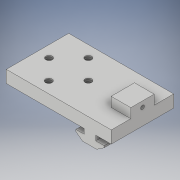
# Autodesk Inventor part: Sliderfor2020
Saved by Autodesk Inventor 2017 (Build 210142000, 142)
## iProperties
Created: 2017-12-08
Part Number: Sliderfor2020
Material: Generic
Document SubType Name: Modeling
Designer: User
Density: 1 g/cm^3
Appearance: Default
Author: User
Autodesk Inventor part; units mm, degrees
ref_plane "YZ Plane" through (0, 0, 0) normal (1, 0, 0) x (0, 1, 0)
ref_plane "XZ Plane" through (0, 0, 0) normal (0, 1, 0) x (-1, 0, 0)
ref_plane "XY Plane" through (0, 0, 0) normal (0, 0, 1) x (1, 0, 0)
sketch "Sketch1" plane through (0, 0, 0) normal (0, 0, 1) x (1, 0, 0)
  line L0 (0, 0) -> (14.5304, 0)
  line L1 (-8.7854, 6.6412) -> (8.5466, 6.6412)
  line L2 (8.5466, 1.6412) -> (2.2606, 1.6412)
  line L3 (2.2606, 1.6412) -> (2.2606, -0.3588)
  line L4 (2.2606, -0.3588) -> (5.6256, -0.3588)
  line L5 (2.5721, -3.1588) -> (-3.1429, -3.1588)
  line L6 (-3.1429, -3.1588) -> (-5.8644, -1.1208)
  line L7 (-5.8644, -1.1208) -> (-5.8644, -0.3588)
  line L8 (-5.8644, -0.3588) -> (-2.4994, -0.3588)
  line L9 (-2.4994, -0.3588) -> (-2.4994, 1.6412)
  line L10 (-2.4994, 1.6412) -> (-8.7854, 1.6412)
  line L11 (-8.7854, 1.6412) -> (-8.7854, 6.6412)
  line L12 (5.6256, -0.3588) -> (5.6256, -1.1208)
  line L13 (5.6256, -1.1208) -> (2.5721, -3.1588)
  line L14 (8.5466, 6.6412) -> (5.0156, 6.6412)
  line L15 (5.0156, 1.6412) -> (8.5466, 1.6412)
  line L16 (8.5466, 6.6412) -> (8.5466, 1.6412)
  dimension "d2" = 5
  dimension "d3" = 2
  dimension "d6" = 11.49
  dimension "d7" = 2.921
  dimension "d9" = 5.6425
  dimension "d11" = 0.762
  dimension "d12" = 0.762
  dimension "d78" = 2.921
  dimension "d88" = 3.365
  dimension "d89" = 3.365
  constraints: 34 end point, 5 perpendicular, 4 point on line, 3 horizontal, 2 vertical, 1 collinear
  measures "d2" distance between parallel lines of L10 L1
  measures "d3" distance between parallel lines of L8 L10
  measures "d6" distance between parallel lines of L7 L12
  measures "d7" distance between parallel lines of L7 L11
  measures "d9" distance from line of L5.end L11
  measures "d11" distance of L6.end L7.end
  measures "d12" distance of L4.end L12.end
  measures "d78" distance between parallel lines of L16 L12
  measures "d88" distance between parallel lines of L9 L7
  measures "d89" distance from line of L4.end L3
extrude "Extrusion1" add sketch "Sketch1" along normal blind 25.4
sketch "Sketch4" plane through (8.5466, 1.6412, 0) normal (1, 0, 0) x (0, 0, -1)
  line L0 (0, 5) -> (0, 0) projected
  line L1 (0, 5) -> (-25.4, 5) projected
  line L2 (-25.4, 0) -> (-25.4, 5) projected
  line L3 (0, 0) -> (-25.4, 0) projected
  line L4 (-12.7, 0) -> (-19.05, 0)
  line L5 (0, 0) -> (-25.4, 0) projected
  line L6 (-7.9375, 0) -> (-17.4625, 0)
  line L7 (-17.4625, 0) -> (-17.4625, 8.89)
  line L8 (-17.4625, 8.89) -> (-7.9375, 8.89)
  line L9 (-7.9375, 8.89) -> (-7.9375, 0)
  point P0 (0, -1.6412)
  dimension "d40" = 25.4
  dimension "d41" = 9.525
  dimension "d42" = 8.89
  dimension "d43" = 7.9375
  constraints: 10 end point, 2 horizontal, 2 parallel, 1 midpoint, 1 perpendicular, 1 point on line
  measures "d40" distance of L0.start L1.end
  measures "d41" distance of L7.end L8.end
  measures "d42" distance of L6.end L7.end
  measures "d43" distance between parallel lines of L0 L9
extrude "Extrusion3" add sketch "Sketch4" against normal blind 8 contours L9 L3 L7 L1 | L1 L7 L8 L9
sketch "Sketch6" plane through (8.5466, 1.6412, 0) normal (1, 0, 0) x (0, 0, -1)
  line L0 (0, 0) -> (-25.4, 0) projected
  line L1 (-7.9375, 8.89) -> (-17.4625, 8.89) projected
  line L2 (-25.4, 0) -> (-25.4, 5) projected
  line L3 (0, 5) -> (0, 0) projected
  circle A0 centre (-12.7, 6.604) radius 1.5
  point P0 (0, -1.6412)
  dimension "d46" = 8.89
  dimension "d47" = 25.4
  dimension "d50" = 3
  dimension "d58" = 6.604
  dimension "d59" = 12.7
  constraints: 1 centre point, 1 coincident
  measures "d46" distance between parallel lines of L0 L1
  measures "d47" distance between parallel lines of L2 L3
  measures "d50" diameter of A0
  measures "d58" distance from line of L0 A0.centre
  measures "d59" distance from line of L2 A0.centre
hole "Hole2" at (8.5466, 8.2452, 12.7) direction (-1, 0, 0) diameter 1.5748 end through all
sketch "Sketch7" plane through (-8.7854, 1.6412, 0) normal (-1, 0, 0) x (0, 0, 1)
  line L0 (0, 0) -> (0, 5) projected
  line L1 (0, 0) -> (25.4, 0) projected
  line L2 (25.4, 5) -> (25.4, 0) projected
  line L3 (0, 5) -> (25.4, 5) projected
  point P0 (0, -1.6412)
extrude "Extrusion4" add sketch "Sketch7" along normal blind 25.4
sketch "Sketch9" plane through (0.5466, 6.6412, 7.9375) normal (0, 1, 0) x (1, 0, 0)
  circle A0 centre (-19.2542, -4.7625) radius 1.3208 projected
  line L0 (-9.332, 3.2385) -> (-22.032, 3.2385)
  line L1 (-17.333, -4.7625) -> (-30.033, -4.7625)
  line L2 (-1.331, -4.7625) -> (-14.031, -4.7625)
  line L3 (-9.332, -12.8819) -> (-22.032, -12.8819)
  circle A1 centre (-22.032, -4.7625) radius 8.001
  line L4 (-34.732, -17.4625) -> (-34.732, 7.9375) projected
  line L5 (-34.732, 7.9375) -> (8, 7.9375) projected
  point P0 (-0.5466, 7.9375)
  dimension "d101" = 12.7
  dimension "d102" = 12.7
  dimension "d103" = 12.7
  dimension "d104" = 12.7
  dimension "d112" = 12.7
  dimension "d113" = 16.002
  dimension "d114" = 25.4
  dimension "d115" = 12.7
  constraints: 8 end point, 4 coincident, 4 horizontal, 3 point on circle, 1 centre point, 1 point on line, 1 tangent
  measures "d101" distance of L0.start L0.end
  measures "d102" distance of L1.start L1.end
  measures "d103" distance of L2.start L2.end
  measures "d104" distance of L3.start L3.end
  measures "d112" distance from line of L4 A1.centre
  measures "d113" diameter of A1
  measures "d114" distance of L4.start L4.end
  measures "d115" distance from line of L5 A1.centre
hole "Hole5" at (-13.4844, 6.6412, 12.7) at (-21.4854, 6.6412, 4.699) at (-29.4864, 6.6412, 12.7) at (-21.4854, 6.6412, 20.8194) direction (0, -1, 0) diameter 2.6416 end through all thread size "6-32 UNC" class "2B" standard "ANSI Unified Screw Threads"
equation "\"d9\" = -0.5 * d8 + 0.5 * d0"
equation "\"d12\" = d11"
equation "\"d43\" = -0.5 * d41 + 0.5 * d40"
equation "\"d59\" = 0.5 * d47"
equation "\"d115\" = 0.5 * d114"
equation "\"d8\" = 5.715"
equation "\"d0\" = 17"
body "Solid1"
